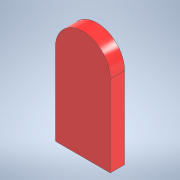
# Autodesk Inventor part: rgb led
Saved by Autodesk Inventor 2021 (Build 250183000, 183)
## iProperties
Created: 2021-07-28
Part Number: rgb led
Material: Generic
Document SubType Name: Modeling
Designer: Dell
Density: 1 g/cm^3
Appearance: Default
Author: Dell
Autodesk Inventor part; units mm, degrees
ref_plane "YZ Plane" through (0, 0, 0) normal (1, 0, 0) x (0, 1, 0)
ref_plane "XZ Plane" through (0, 0, 0) normal (0, 1, 0) x (-1, 0, 0)
ref_plane "XY Plane" through (0, 0, 0) normal (0, 0, 1) x (1, 0, 0)
sketch "Sketch1" plane through (0, 0, 0) normal (0, 0, 1) x (1, 0, 0)
  line L0 (-8.0598, 3.2108) -> (-6.094, 3.2108) construction
  spline S0 degree 1 poles (-8.0598, 3.2108) (-6.094, 3.2108) knots 1 1 2 2
  line L1 (-8.0162, 3.2982) -> (-8.0162, 5.4824) construction
  spline S1 degree 1 poles (-8.0162, 3.2982) (-8.0162, 5.4824) knots 1 1 2 2
  line L2 (-6.094, 3.2108) -> (-6.094, 5.4824) construction
  spline S2 degree 1 poles (-6.094, 3.2108) (-6.094, 5.4824) knots 1 1 2 2
  circle A0 centre (-7.0769, 5.4824) radius 0.9573
  point P0 (0, 0)
  constraints: 1 centre point, 1 horizontal, 1 vertical, 9 other
extrude "Extrusion1" add sketch "Sketch1" along normal blind 0.5
sketch "Sketch2" plane through (-7.0769, 5.4824, 0.5) normal (0, 0, 1) x (1, 0, 0)
  circle A0 centre (0, 0) radius 0.9573 projected
  line L0 (-0.9573, 0) -> (-0.9573, -2.8395) construction
  spline S0 degree 1 poles (-0.9573, 0) (-0.9573, -2.8395) knots 1 1 2 2
  line L1 (0.9573, 0) -> (0.9573, -2.8395) construction
  spline S1 degree 1 poles (0.9573, 0) (0.9573, -2.8395) knots 1 1 2 2
  line L2 (-0.9573, -2.8395) -> (0.9573, -2.8395) construction
  spline S2 degree 1 poles (-0.9573, -2.8395) (0.9573, -2.8395) knots 1 1 2 2
  line L3 (-0.9573, -2.8395) -> (0, -2.8395) construction
  spline S3 degree 1 poles (-0.9573, -2.8395) (0, -2.8395) knots 1 1 2 2
  point P0 (7.0769, -5.4824)
  constraints: 2 point on circle, 2 tangent, 2 vertical, 1 horizontal, 13 other
extrude "Extrusion2" add sketch "Sketch2" against normal blind 0.5 contours S1 S2 S0 A0
body "Solid1"
